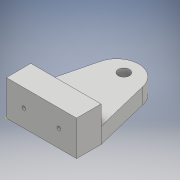
# Autodesk Inventor part: upper_deck_shaft_mount
Saved by Autodesk Inventor 2017 (Build 210142000, 142)
## iProperties
Created: 2017-08-21
Part Number: upper_deck_shaft_mount
Material: Generic
Document SubType Name: Modeling
Designer: ndz
Density: 1 g/cm^3
Appearance: Default
Author: ndz
Autodesk Inventor part; units mm, degrees
ref_plane "YZ Plane" through (0, 0, 0) normal (1, 0, 0) x (0, 1, 0)
ref_plane "XZ Plane" through (0, 0, 0) normal (0, 1, 0) x (-1, 0, 0)
ref_plane "XY Plane" through (0, 0, 0) normal (0, 0, 1) x (1, 0, 0)
sketch "Sketch1" plane through (0, 0, 0) normal (0, 0, 1) x (1, 0, 0)
  circle A0 centre (10, 23.5) radius 1.6
  line L0 (-0.0511, 6.9998) -> (3.884, 22.9404)
  line L1 (20, 6.9998) -> (16.1838, 22.6325)
  arc A1 (16.1838, 22.6325) -> (3.884, 22.9404) centre (10, 21.4305) ccw
  line L2 (0, 0) -> (20, 0)
  line L3 (20, 6.9998) -> (16.1838, 22.6325)
  line L4 (0, 0) -> (-0.0511, 6.9998)
  line L5 (20, 0) -> (20, 6.9998)
  dimension "d17" = 7
  dimension "d18" = 6.9998
  constraints: 12 end point, 2 centre point, 2 point on circle, 1 tangent, 1 vertical
  measures "d17" distance of L2.start L0.start
  measures "d18" distance of L2.end L1.start
sketch "Sketch3" plane through (0, 0, 0) normal (0, 0, 1) x (1, 0, 0)
  point P0 (0, 0)
extrude "Extrusion1" add sketch "Sketch1" along normal blind 4.5
sketch "Sketch4" plane through (0, 0, 4.5) normal (0, 0, 1) x (1, 0, 0)
  line L0 (-0.0511, 6.9998) -> (0, 0) projected
  line L1 (20, 0) -> (20, 6.9998) projected
  line L2 (0, 0) -> (20, 0)
  line L3 (20, 0) -> (20, 6.9998)
  line L4 (3.884, 22.9404) -> (-0.0511, 6.9998) projected
  line L5 (20, 6.9998) -> (-0.0511, 6.9998)
  line L6 (0, 6.9998) -> (0, 0)
  constraints: 8 end point, 3 perpendicular, 1 collinear
extrude "Extrusion2" add sketch "Sketch4" along normal blind 5.5
sketch "Sketch5" plane through (0, 0, 0) normal (0, -1, 0) x (1, 0, 0)
  circle A0 centre (5, 5) radius 0.5
  circle A1 centre (15, 5) radius 0.5
  point P0 (0, 0)
  dimension "d13" = 1
  dimension "d14" = 1
  constraints: 2 centre point
  measures "d13" diameter of A0
  measures "d14" diameter of A1
extrude "Extrusion3" cut sketch "Sketch5" against normal blind 5.5
body "Solid1"
